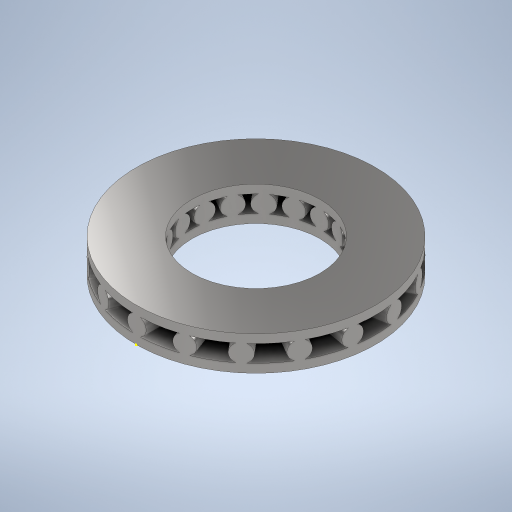
# Autodesk Inventor part: AXK1528+AS Bearing
Saved by Autodesk Inventor 2024.1 (Build 281209000, 209)
## iProperties
Created: 2023-09-08
Part Number: AXK1528+AS Bearing
Material: Stainless Steel
Document SubType Name: Modeling
Designer: chanh
Density: 8 g/cm^3
Appearance: Semi-Polished
Author: chanh
Autodesk Inventor part; units mm, degrees
ref_plane "YZ Plane" through (0, 0, 0) normal (1, 0, 0) x (0, 1, 0)
sketch "Sketch1" plane through (0, 0, 0) normal (0, 1, 0) x (-1, 0, 0)
  circle A0 centre (0, 0) radius 14
  circle A1 centre (0, 0) radius 7.5
  dimension "d0" = 28
  dimension "d1" = 15
  constraints: 2 centre point, 2 coincident
  measures "d0" diameter of A0
  measures "d1" diameter of A1
extrude "Extrusion1" add sketch "Sketch1" along normal blind 1
ref_plane "Work Plane1" through (0, 0, 14) normal (0, 0, 1) x (1, 0, 0)
sketch "Sketch2" plane through (0, 0, 14) normal (0, 0, 1) x (1, 0, 0)
  line L0 (14, 1) -> (-14, 1) projected
  circle A0 centre (0, 2) radius 1.1
  point P0 (0, 0)
  point P1 (0.4583, 1)
  point P2 (-0.4583, 1)
  dimension "d4" = 2.2
  dimension "d5" = 2
  constraints: 1 centre point, 1 vertical alignment
  measures "d4" diameter of A0
  measures "d5" distance of A0.centre point (0, 0)
extrude "Extrusion2" add sketch "Sketch2" against normal blind 11.5875 contours L0 A0 picked at (0.3793, 1.7905)
pattern_circular "Circular Pattern1" count 18 over 360 about axis through (0, -10, 0) along (0, 1, 0) of "Extrusion2"
sketch "Sketch3" plane through (0, 0, 14) normal (0, 0, 1) x (1, 0, 0)
  point P0 (0, 0)
ref_plane "Work Plane3" through (0, 3, 14) normal (0, 1, 0) x (1, 0, 0)
ref_plane "Work Plane2" through (0, 3.1, 14) normal (0, 1, 0) x (1, 0, 0)
sketch "Sketch4" plane through (0, 3, 14) normal (0, 1, 0) x (1, 0, 0)
  circle A0 centre (0, 14) radius 7.5 projected
  circle A1 centre (0, 14) radius 14 projected
extrude "Extrusion3" add sketch "Sketch4" along normal blind 1
sketch "Sketch5" plane through (0, 4, 0) normal (0, 1, 0) x (1, 0, 0)
  circle A0 centre (0, 0) radius 7.5 projected
  circle A1 centre (0, 0) radius 14 projected
  circle A2 centre (0, 0) radius 19
  dimension "d14" = 5
  constraints: 1 centre point
  measures "d14" radial gap between concentric circles of A1 A2
extrude "Extrusion4" cut sketch "Sketch5" against normal through all
body "Solid1"
